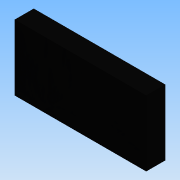
# Autodesk Inventor part: speaker
Saved by Autodesk Inventor 2015 (Build 190159000, 159)
## iProperties
Created: 2016-04-19
Part Number: speaker
Material: Générique
Document SubType Name: Modeling
Designer: Gregwar
Density: 1 g/cm^3
Appearance: Par défaut
Author: Gregwar
Autodesk Inventor part; units mm, degrees
ref_plane "YZ Plane" through (0, 0, 0) normal (1, 0, 0) x (0, 1, 0)
ref_plane "XZ Plane" through (0, 0, 0) normal (0, 1, 0) x (-1, 0, 0)
ref_plane "XY Plane" through (0, 0, 0) normal (0, 0, 1) x (1, 0, 0)
sketch "Esquisse1" plane through (0, 0, 0) normal (0, 1, 0) x (-1, 0, 0)
  line L0 (0, 0) -> (40, 0)
  line L1 (40, 0) -> (40, -20)
  line L2 (40, -20) -> (0, -20)
  line L3 (0, -20) -> (0, 0)
  dimension "d0" = 20
  dimension "d1" = 40
  constraints: 8 end point, 2 parallel, 1 horizontal, 1 perpendicular
  measures "d0" distance of L2.end L0.start
  measures "d1" distance of L0.start L0.end
extrude "Extrusion1" add sketch "Esquisse1" along normal blind 5.8
